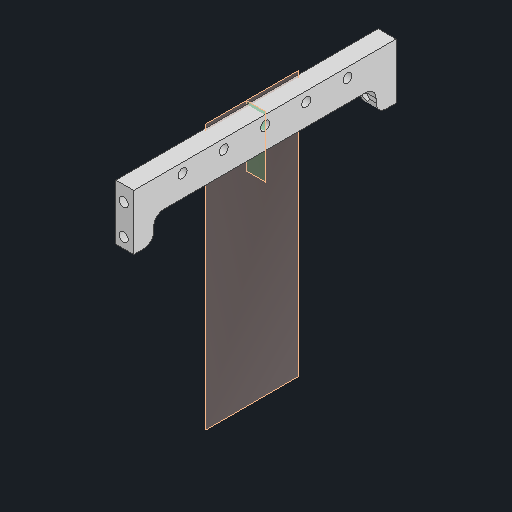
# Autodesk Inventor part: pci_slot_adapter_01
Saved by Autodesk Inventor 2022 (Build 260153000, 153)
## iProperties
Created: 2025-02-02
Part Number: pci_slot_adapter_01
Material: 一般
Document SubType Name: Modeling
Designer: nyxeon
Density: 1 g/cm^3
Appearance: 既定
Author: nyxeon
Autodesk Inventor part; units mm, degrees
ref_plane "YZ Plane" through (0, 0, 0) normal (1, 0, 0) x (0, 1, 0)
ref_plane "XZ Plane" through (0, 0, 0) normal (0, 1, 0) x (-1, 0, 0)
ref_plane "XY Plane" through (0, 0, 0) normal (0, 0, 1) x (1, 0, 0)
ref_plane "作業平面1" through (247.124, 159, 65.625) normal (1, 0, 0) x (0, 1, 0)
sketch "スケッチ1" plane through (247.124, 159, 65.625) normal (1, 0, 0) x (0, 1, 0)
  line L0 (60.3482, -6.7165) -> (60.3482, -14.8665) construction
  arc A0 (59.1658, -16) -> (60.3482, -14.8665) centre (59.15, -14.8001) ccw construction
  line L1 (53.4901, -16) -> (59.1658, -16) construction
  arc A1 (53.4901, -16) -> (53.2698, -16.0957) centre (53.4895, -16.3) ccw construction
  arc A2 (60.3482, -6.7165) -> (59.15, -5.583) centre (59.15, -6.783) ccw construction
  line L2 (59.15, -5.583) -> (53.4743, -5.583) construction
  line L3 (53.2621, -5.4951) -> (49.3015, -1.5345) construction
  arc A3 (53.2621, -5.4951) -> (53.4743, -5.583) centre (53.4743, -5.283) ccw construction
  arc A4 (48.95, -0.6859) -> (49.3015, -1.5345) centre (50.15, -0.6859) ccw construction
  arc A5 (49.3015, 0.2515) -> (48.95, -0.5971) centre (50.15, -0.5971) ccw construction
  line L4 (48.95, -0.6859) -> (48.95, -0.5971) construction
  line L5 (49.3015, 0.2515) -> (53.2621, 4.2121) construction
  arc A6 (53.4743, 4.3) -> (53.2621, 4.2121) centre (53.4743, 4) ccw construction
  line L6 (53.4743, 4.3) -> (59.15, 4.3) construction
  arc A7 (59.15, 4.3) -> (60.35, 5.5) centre (59.15, 5.5) ccw construction
  line L7 (60.35, 13.65) -> (60.35, 5.5) construction
  arc A8 (60.35, 13.65) -> (59.15, 14.85) centre (59.15, 13.65) ccw construction
  line L8 (59.15, 14.85) -> (53.4743, 14.85) construction
  arc A9 (53.2621, 14.9379) -> (53.4743, 14.85) centre (53.4743, 15.15) ccw construction
  line L9 (58.1, -68.625) -> (53.9, -68.625) construction
  line L10 (43.1, -68.625) -> (38.9, -68.625) construction
  line L11 (41, -68.625) -> (41, 67.375) construction
  line L12 (56, -68.625) -> (56, 67.375) construction
  line L13 (60.3482, -10.7915) -> (50.15, -10.7915) construction
  line L14 (60.35, 9.575) -> (50.15, 9.575) construction
  arc A10 (49.3015, -20.0486) -> (48.95, -20.8972) centre (50.15, -20.8972) ccw construction
  arc A11 (48.95, -20.986) -> (49.3015, -21.8346) centre (50.15, -20.986) ccw construction
  line L15 (48.95, -20.8972) -> (48.95, -20.986) construction
  line L16 (53.2698, -16.0957) -> (49.3015, -20.0486) construction
  line L17 (60.3482, 25.8665) -> (60.3482, 34.0165) construction
  arc A12 (60.3482, 34.0165) -> (59.1658, 35.15) centre (59.15, 33.9501) ccw construction
  line L18 (53.4901, 35.15) -> (59.1658, 35.15) construction
  arc A13 (53.2698, 35.2457) -> (53.4901, 35.15) centre (53.4895, 35.45) ccw construction
  arc A14 (59.15, 24.733) -> (60.3482, 25.8665) centre (59.15, 25.933) ccw construction
  line L19 (59.15, 24.733) -> (53.4743, 24.733) construction
  line L20 (53.2621, 24.6451) -> (49.3015, 20.6845) construction
  arc A15 (53.4743, 24.733) -> (53.2621, 24.6451) centre (53.4743, 24.433) ccw construction
  arc A16 (49.3015, 20.6845) -> (48.95, 19.8359) centre (50.15, 19.8359) ccw construction
  arc A17 (48.95, 19.7471) -> (49.3015, 18.8985) centre (50.15, 19.7471) ccw construction
  line L21 (48.95, 19.8359) -> (48.95, 19.7471) construction
  line L22 (49.3015, 18.8985) -> (53.2621, 14.9379) construction
  arc A18 (48.95, 40.0472) -> (49.3015, 39.1986) centre (50.15, 40.0472) ccw construction
  arc A19 (49.3015, 40.9846) -> (48.95, 40.136) centre (50.15, 40.136) ccw construction
  line L23 (48.95, 40.0472) -> (48.95, 40.136) construction
  line L24 (53.2698, 35.2457) -> (49.3015, 39.1986) construction
  line L25 (60.3482, 29.9415) -> (50.15, 29.9415) construction
  line L26 (60.3482, 66.5996) -> (60.3482, 74.7496) construction
  arc A20 (60.3482, 74.7496) -> (59.1658, 75.8831) centre (59.15, 74.6832) ccw construction
  line L27 (53.4901, 75.8831) -> (59.1658, 75.8831) construction
  arc A21 (53.2698, 75.9787) -> (53.4901, 75.8831) centre (53.4895, 76.1831) ccw construction
  arc A22 (59.15, 65.4661) -> (60.3482, 66.5996) centre (59.15, 66.6661) ccw construction
  line L28 (59.15, 65.4661) -> (53.4743, 65.4661) construction
  line L29 (53.2621, 65.3782) -> (49.3015, 61.4175) construction
  arc A23 (53.4743, 65.4661) -> (53.2621, 65.3782) centre (53.4743, 65.1661) ccw construction
  arc A24 (49.3015, 61.4175) -> (48.95, 60.569) centre (50.15, 60.569) ccw construction
  arc A25 (48.95, 60.4801) -> (49.3015, 59.6316) centre (50.15, 60.4801) ccw construction
  line L30 (48.95, 60.569) -> (48.95, 60.4801) construction
  line L31 (49.3015, 59.6316) -> (53.2621, 55.671) construction
  arc A26 (53.2621, 55.671) -> (53.4743, 55.5831) centre (53.4743, 55.8831) ccw construction
  line L32 (53.4743, 55.5831) -> (59.15, 55.5831) construction
  arc A27 (60.35, 54.3831) -> (59.15, 55.5831) centre (59.15, 54.3831) ccw construction
  line L33 (60.35, 46.2331) -> (60.35, 54.3831) construction
  arc A28 (59.15, 45.0331) -> (60.35, 46.2331) centre (59.15, 46.2331) ccw construction
  line L34 (59.15, 45.0331) -> (53.4743, 45.0331) construction
  arc A29 (53.4743, 45.0331) -> (53.2621, 44.9452) centre (53.4743, 44.7331) ccw construction
  arc A30 (48.95, 80.7802) -> (49.3015, 79.9317) centre (50.15, 80.7802) ccw construction
  arc A31 (49.3015, 81.7176) -> (48.95, 80.8691) centre (50.15, 80.8691) ccw construction
  line L35 (48.95, 80.7802) -> (48.95, 80.8691) construction
  line L36 (53.2698, 75.9787) -> (49.3015, 79.9317) construction
  line L37 (49.3015, 40.9846) -> (53.2621, 44.9452) construction
  line L38 (49.3015, -21.8346) -> (53.2621, -25.7952) construction
  arc A32 (53.2621, -25.7952) -> (53.4743, -25.8831) centre (53.4743, -25.5831) ccw construction
  line L39 (53.4743, -25.8831) -> (59.15, -25.8831) construction
  arc A33 (60.35, -27.0831) -> (59.15, -25.8831) centre (59.15, -27.0831) ccw construction
  line L40 (60.35, -35.2331) -> (60.35, -27.0831) construction
  arc A34 (59.15, -36.4331) -> (60.35, -35.2331) centre (59.15, -35.2331) ccw construction
  line L41 (59.15, -36.4331) -> (53.4743, -36.4331) construction
  arc A35 (53.4743, -36.4331) -> (53.2621, -36.521) centre (53.4743, -36.7331) ccw construction
  line L42 (49.3015, -40.4816) -> (53.2621, -36.521) construction
  arc A36 (49.3015, -40.4816) -> (48.95, -41.3301) centre (50.15, -41.3301) ccw construction
  line L43 (48.95, -41.419) -> (48.95, -41.3301) construction
  arc A37 (48.95, -41.419) -> (49.3015, -42.2675) centre (50.15, -41.419) ccw construction
  line L44 (53.2621, -46.2282) -> (49.3015, -42.2675) construction
  arc A38 (53.2621, -46.2282) -> (53.4743, -46.3161) centre (53.4743, -46.0161) ccw construction
  line L45 (59.15, -46.3161) -> (53.4743, -46.3161) construction
  arc A39 (60.3482, -47.4496) -> (59.15, -46.3161) centre (59.15, -47.5161) ccw construction
  line L46 (60.3482, -47.4496) -> (60.3482, -55.5996) construction
  arc A40 (59.1658, -56.7331) -> (60.3482, -55.5996) centre (59.15, -55.5332) ccw construction
  line L47 (53.4901, -56.7331) -> (59.1658, -56.7331) construction
  arc A41 (53.4901, -56.7331) -> (53.2698, -56.8287) centre (53.4895, -57.0331) ccw construction
  line L48 (53.2698, -56.8287) -> (49.3015, -60.7817) construction
  arc A42 (49.3015, -60.7817) -> (48.95, -61.6302) centre (50.15, -61.6302) ccw construction
  line L49 (48.95, -61.6302) -> (48.95, -61.7191) construction
  arc A43 (48.95, -61.7191) -> (49.3015, -62.5676) centre (50.15, -61.7191) ccw construction
  line L50 (49.3015, -62.5676) -> (53.2621, -66.5283) construction
  arc A44 (53.2621, -66.5283) -> (53.4743, -66.6162) centre (53.4743, -66.3162) ccw construction
  line L51 (59.15, -66.6162) -> (53.4743, -66.6162) construction
  arc A45 (60.35, -67.8162) -> (59.15, -66.6162) centre (59.15, -67.8162) ccw construction
  line L52 (60.35, -67.8162) -> (60.35, -75.9662) construction
  arc A46 (59.15, -77.1662) -> (60.35, -75.9662) centre (59.15, -75.9662) ccw construction
  line L53 (53.4743, -77.1662) -> (59.15, -77.1662) construction
  arc A47 (53.4743, -77.1662) -> (53.2621, -77.254) centre (53.4743, -77.4662) ccw construction
  line L54 (49.3015, -81.2147) -> (53.2621, -77.254) construction
  arc A48 (49.3015, -81.2147) -> (48.95, -82.0632) centre (50.15, -82.0632) ccw construction
  line L55 (48.95, -82.1521) -> (48.95, -82.0632) construction
  arc A49 (48.95, -82.1521) -> (49.3015, -83.0006) centre (50.15, -82.1521) ccw construction
  line L56 (53.2621, -86.9613) -> (49.3015, -83.0006) construction
  arc A50 (49.4429, 81.5762) -> (49.15, 80.8691) centre (50.15, 80.8691) ccw
  line L57 (49.15, 80.8691) -> (49.15, 80.7802)
  arc A51 (49.15, 80.7802) -> (49.4443, 80.0718) centre (50.15, 80.7802) ccw
  line L58 (49.4443, 80.0718) -> (53.4144, 76.117)
  arc A52 (53.4144, 76.117) -> (53.4897, 76.0831) centre (53.4895, 76.1831) ccw
  line L59 (53.4897, 76.0831) -> (59.1671, 76.0831)
  arc A53 (60.5482, 74.755) -> (59.1671, 76.0831) centre (59.15, 74.6832) ccw
  line L60 (60.5482, 74.755) -> (60.5482, 66.7378)
  arc A54 (59.15, 65.2661) -> (60.5482, 66.7378) centre (59.15, 66.6661) ccw
  line L61 (59.15, 65.2661) -> (53.4743, 65.2661)
  arc A55 (53.4743, 65.2661) -> (53.4036, 65.2368) centre (53.4743, 65.1661) ccw
  line L62 (53.4036, 65.2368) -> (49.4429, 61.2761)
  arc A56 (49.4429, 61.2761) -> (49.15, 60.569) centre (50.15, 60.569) ccw
  line L63 (49.15, 60.569) -> (49.15, 60.4801)
  arc A57 (49.15, 60.4801) -> (49.4429, 59.773) centre (50.15, 60.4801) ccw
  line L64 (49.4429, 59.773) -> (53.4036, 55.8124)
  arc A58 (53.4036, 55.8124) -> (53.4743, 55.7831) centre (53.4743, 55.8831) ccw
  line L65 (53.4743, 55.7831) -> (59.15, 55.7831)
  arc A59 (60.55, 54.3831) -> (59.15, 55.7831) centre (59.15, 54.3831) ccw
  line L66 (60.55, 54.3831) -> (60.55, 46.2331)
  arc A60 (59.15, 44.8331) -> (60.55, 46.2331) centre (59.15, 46.2331) ccw
  line L67 (59.15, 44.8331) -> (53.4743, 44.8331)
  arc A61 (53.4743, 44.8331) -> (53.4036, 44.8038) centre (53.4743, 44.7331) ccw
  line L68 (53.4036, 44.8038) -> (49.4429, 40.8431)
  arc A62 (49.4429, 40.8431) -> (49.15, 40.136) centre (50.15, 40.136) ccw
  line L69 (49.15, 40.136) -> (49.15, 40.0472)
  arc A63 (49.15, 40.0472) -> (49.4443, 39.3387) centre (50.15, 40.0472) ccw
  line L70 (49.4443, 39.3387) -> (53.4144, 35.384)
  arc A64 (53.4144, 35.384) -> (53.4897, 35.35) centre (53.4895, 35.45) ccw
  line L71 (53.4897, 35.35) -> (59.1671, 35.35)
  arc A65 (60.5482, 34.0219) -> (59.1671, 35.35) centre (59.15, 33.9501) ccw
  line L72 (60.5482, 34.0219) -> (60.5482, 26.0047)
  arc A66 (59.15, 24.533) -> (60.5482, 26.0047) centre (59.15, 25.933) ccw
  line L73 (59.15, 24.533) -> (53.4743, 24.533)
  arc A67 (53.4743, 24.533) -> (53.4036, 24.5037) centre (53.4743, 24.433) ccw
  line L74 (53.4036, 24.5037) -> (49.4429, 20.543)
  arc A68 (49.4429, 20.543) -> (49.15, 19.8359) centre (50.15, 19.8359) ccw
  line L75 (49.15, 19.8359) -> (49.15, 19.7471)
  arc A69 (49.15, 19.7471) -> (49.4429, 19.0399) centre (50.15, 19.7471) ccw
  line L76 (49.4429, 19.0399) -> (53.4036, 15.0793)
  arc A70 (53.4036, 15.0793) -> (53.4743, 15.05) centre (53.4743, 15.15) ccw
  line L77 (53.4743, 15.05) -> (59.15, 15.05)
  arc A71 (60.55, 13.65) -> (59.15, 15.05) centre (59.15, 13.65) ccw
  line L78 (60.55, 13.65) -> (60.55, 5.5)
  arc A72 (59.15, 4.1) -> (60.55, 5.5) centre (59.15, 5.5) ccw
  line L79 (59.15, 4.1) -> (53.4743, 4.1)
  arc A73 (53.4743, 4.1) -> (53.4036, 4.0707) centre (53.4743, 4) ccw
  line L80 (53.4036, 4.0707) -> (49.4429, 0.1101)
  arc A74 (49.4429, 0.1101) -> (49.15, -0.5971) centre (50.15, -0.5971) ccw
  line L81 (49.15, -0.5971) -> (49.15, -0.6859)
  arc A75 (49.15, -0.6859) -> (49.4429, -1.393) centre (50.15, -0.6859) ccw
  line L82 (49.4429, -1.393) -> (53.4036, -5.3537)
  arc A76 (53.4036, -5.3537) -> (53.4743, -5.383) centre (53.4743, -5.283) ccw
  line L83 (53.4743, -5.383) -> (59.15, -5.383)
  arc A77 (60.5482, -6.8547) -> (59.15, -5.383) centre (59.15, -6.783) ccw
  line L84 (60.5482, -6.8547) -> (60.5482, -14.8719)
  arc A78 (59.1671, -16.2) -> (60.5482, -14.8719) centre (59.15, -14.8001) ccw
  line L85 (59.1671, -16.2) -> (53.4897, -16.2)
  arc A79 (53.4897, -16.2) -> (53.4144, -16.234) centre (53.4895, -16.3) ccw
  line L86 (53.4144, -16.234) -> (49.4443, -20.1887)
  arc A80 (49.4443, -20.1887) -> (49.15, -20.8972) centre (50.15, -20.8972) ccw
  line L87 (49.15, -20.8972) -> (49.15, -20.986)
  arc A81 (49.15, -20.986) -> (49.4429, -21.6931) centre (50.15, -20.986) ccw
  line L88 (49.4429, -21.6931) -> (53.4036, -25.6538)
  arc A82 (53.4036, -25.6538) -> (53.4743, -25.6831) centre (53.4743, -25.5831) ccw
  line L89 (53.4743, -25.6831) -> (59.15, -25.6831)
  arc A83 (60.55, -27.0831) -> (59.15, -25.6831) centre (59.15, -27.0831) ccw
  line L90 (60.55, -27.0831) -> (60.55, -35.2331)
  arc A84 (59.15, -36.6331) -> (60.55, -35.2331) centre (59.15, -35.2331) ccw
  line L91 (59.15, -36.6331) -> (53.4743, -36.6331)
  arc A85 (53.4743, -36.6331) -> (53.4036, -36.6624) centre (53.4743, -36.7331) ccw
  line L92 (53.4036, -36.6624) -> (49.4429, -40.623)
  arc A86 (49.4429, -40.623) -> (49.15, -41.3301) centre (50.15, -41.3301) ccw
  line L93 (49.15, -41.3301) -> (49.15, -41.419)
  arc A87 (49.15, -41.419) -> (49.4429, -42.1261) centre (50.15, -41.419) ccw
  line L94 (49.4429, -42.1261) -> (53.4036, -46.0868)
  arc A88 (53.4036, -46.0868) -> (53.4743, -46.1161) centre (53.4743, -46.0161) ccw
  line L95 (53.4743, -46.1161) -> (59.15, -46.1161)
  arc A89 (60.5482, -47.5878) -> (59.15, -46.1161) centre (59.15, -47.5161) ccw
  line L96 (60.5482, -47.5878) -> (60.5482, -55.605)
  arc A90 (59.1671, -56.9331) -> (60.5482, -55.605) centre (59.15, -55.5332) ccw
  line L97 (59.1671, -56.9331) -> (53.4897, -56.9331)
  arc A91 (53.4897, -56.9331) -> (53.4144, -56.967) centre (53.4895, -57.0331) ccw
  line L98 (53.4144, -56.967) -> (49.4443, -60.9218)
  arc A92 (49.4443, -60.9218) -> (49.15, -61.6302) centre (50.15, -61.6302) ccw
  line L99 (49.15, -61.6302) -> (49.15, -61.7191)
  arc A93 (49.15, -61.7191) -> (49.4429, -62.4262) centre (50.15, -61.7191) ccw
  line L100 (49.4429, -62.4262) -> (53.4036, -66.3869)
  arc A94 (53.4036, -66.3869) -> (53.4743, -66.4162) centre (53.4743, -66.3162) ccw
  line L101 (53.4743, -66.4162) -> (59.15, -66.4162)
  arc A95 (60.55, -67.8162) -> (59.15, -66.4162) centre (59.15, -67.8162) ccw
  line L102 (60.55, -67.8162) -> (60.55, -75.9662)
  arc A96 (59.15, -77.3662) -> (60.55, -75.9662) centre (59.15, -75.9662) ccw
  line L103 (59.15, -77.3662) -> (53.4743, -77.3662)
  arc A97 (53.4743, -77.3662) -> (53.4036, -77.3955) centre (53.4743, -77.4662) ccw
  line L104 (53.4036, -77.3955) -> (49.4429, -81.3561)
  arc A98 (49.4429, -81.3561) -> (49.15, -82.0632) centre (50.15, -82.0632) ccw
  line L105 (49.15, -82.0632) -> (49.15, -82.1521)
  arc A99 (49.15, -82.1521) -> (49.4429, -82.8592) centre (50.15, -82.1521) ccw
  line L106 (49.4429, -82.8592) -> (53.454, -86.8703)
  line L107 (71, -65.625) -> (-359, -65.625) construction
  line L108 (52.6417, -65.625) -> (63.5, -65.625)
  line L109 (63.5, -65.625) -> (63.5, 64.375)
  line L110 (63.5, 64.375) -> (52.5418, 64.375)
  line L111 (71, 67.375) -> (-359, 67.375) construction
  line L112 (-359, 64.375) -> (71, 64.375) construction
  point P0 (-159, -65.625)
  dimension "d0" = 20.3
  dimension "d1" = 0.2
  dimension "d2" = 7.5
  dimension "d38" = 135
  dimension "d39" = 135
  constraints: 208 end point, 190 point on circle, 121 symmetric about line, 95 centre point, 7 vertical alignment, 5 equal length, 5 equal radius, 5 horizontal, 5 midpoint, 5 point on line, 5 tangent, 3 vertical, 139 other
  measures "d0" distance between parallel lines of L6 L1
  measures "d1" radial gap between concentric circles of A39 A89
  measures "d2" distance between parallel lines of L109 L12
  measures "d38" angle of L79 L80
  measures "d39" angle of L83 L82
extrude "押し出し1" add sketch "スケッチ1" against normal blind 1
sketch "スケッチ2" plane through (247.124, 159, 65.625) normal (1, 0, 0) x (0, 0, -1)
  line L0 (-60.569, 49.15) -> (-60.4801, 49.15) projected
  arc A0 (-60.4801, 49.15) -> (-59.773, 49.4429) centre (-60.4801, 50.15) ccw projected
  line L1 (-59.773, 49.4429) -> (-55.8124, 53.4036) projected
  arc A1 (-55.8124, 53.4036) -> (-55.7831, 53.4743) centre (-55.8831, 53.4743) ccw projected
  line L2 (-55.7831, 53.4743) -> (-55.7831, 59.15) projected
  arc A2 (-54.3831, 60.55) -> (-55.7831, 59.15) centre (-54.3831, 59.15) ccw projected
  line L3 (-54.3831, 60.55) -> (-46.2331, 60.55) projected
  arc A3 (-44.8331, 59.15) -> (-46.2331, 60.55) centre (-46.2331, 59.15) ccw projected
  line L4 (-44.8331, 59.15) -> (-44.8331, 53.4743) projected
  arc A4 (-44.8331, 53.4743) -> (-44.8038, 53.4036) centre (-44.7331, 53.4743) ccw projected
  line L5 (-44.8038, 53.4036) -> (-40.8431, 49.4429) projected
  arc A5 (-40.8431, 49.4429) -> (-40.136, 49.15) centre (-40.136, 50.15) ccw projected
  line L6 (-40.136, 49.15) -> (-40.0472, 49.15) projected
  arc A6 (-40.0472, 49.15) -> (-39.3387, 49.4443) centre (-40.0472, 50.15) ccw projected
  line L7 (-39.3387, 49.4443) -> (-35.384, 53.4144) projected
  arc A7 (-35.384, 53.4144) -> (-35.35, 53.4897) centre (-35.45, 53.4895) ccw projected
  line L8 (-35.35, 53.4897) -> (-35.35, 59.1671) projected
  arc A8 (-34.0219, 60.5482) -> (-35.35, 59.1671) centre (-33.9501, 59.15) ccw projected
  line L9 (-34.0219, 60.5482) -> (-26.0047, 60.5482) projected
  arc A9 (-24.533, 59.15) -> (-26.0047, 60.5482) centre (-25.933, 59.15) ccw projected
  line L10 (-24.533, 59.15) -> (-24.533, 53.4743) projected
  arc A10 (-24.533, 53.4743) -> (-24.5037, 53.4036) centre (-24.433, 53.4743) ccw projected
  line L11 (-24.5037, 53.4036) -> (-20.543, 49.4429) projected
  arc A11 (-20.543, 49.4429) -> (-19.8359, 49.15) centre (-19.8359, 50.15) ccw projected
  line L12 (-19.8359, 49.15) -> (-19.7471, 49.15) projected
  arc A12 (-19.7471, 49.15) -> (-19.0399, 49.4429) centre (-19.7471, 50.15) ccw projected
  line L13 (-19.0399, 49.4429) -> (-15.0793, 53.4036) projected
  arc A13 (-15.0793, 53.4036) -> (-15.05, 53.4743) centre (-15.15, 53.4743) ccw projected
  line L14 (-15.05, 53.4743) -> (-15.05, 59.15) projected
  arc A14 (-13.65, 60.55) -> (-15.05, 59.15) centre (-13.65, 59.15) ccw projected
  line L15 (-13.65, 60.55) -> (-5.5, 60.55) projected
  arc A15 (-4.1, 59.15) -> (-5.5, 60.55) centre (-5.5, 59.15) ccw projected
  line L16 (-4.1, 59.15) -> (-4.1, 53.4743) projected
  arc A16 (-4.1, 53.4743) -> (-4.0707, 53.4036) centre (-4, 53.4743) ccw projected
  line L17 (-4.0707, 53.4036) -> (-0.1101, 49.4429) projected
  arc A17 (-0.1101, 49.4429) -> (0.5971, 49.15) centre (0.5971, 50.15) ccw projected
  line L18 (0.5971, 49.15) -> (0.6859, 49.15) projected
  arc A18 (0.6859, 49.15) -> (1.393, 49.4429) centre (0.6859, 50.15) ccw projected
  line L19 (1.393, 49.4429) -> (5.3537, 53.4036) projected
  arc A19 (5.3537, 53.4036) -> (5.383, 53.4743) centre (5.283, 53.4743) ccw projected
  line L20 (5.383, 53.4743) -> (5.383, 59.15) projected
  arc A20 (6.8547, 60.5482) -> (5.383, 59.15) centre (6.783, 59.15) ccw projected
  line L21 (6.8547, 60.5482) -> (14.8719, 60.5482) projected
  arc A21 (16.2, 59.1671) -> (14.8719, 60.5482) centre (14.8001, 59.15) ccw projected
  line L22 (16.2, 59.1671) -> (16.2, 53.4897) projected
  arc A22 (16.2, 53.4897) -> (16.234, 53.4144) centre (16.3, 53.4895) ccw projected
  line L23 (16.234, 53.4144) -> (20.1887, 49.4443) projected
  arc A23 (20.1887, 49.4443) -> (20.8972, 49.15) centre (20.8972, 50.15) ccw projected
  line L24 (20.8972, 49.15) -> (20.986, 49.15) projected
  arc A24 (20.986, 49.15) -> (21.6931, 49.4429) centre (20.986, 50.15) ccw projected
  line L25 (21.6931, 49.4429) -> (25.6538, 53.4036) projected
  arc A25 (25.6538, 53.4036) -> (25.6831, 53.4743) centre (25.5831, 53.4743) ccw projected
  line L26 (25.6831, 53.4743) -> (25.6831, 59.15) projected
  arc A26 (27.0831, 60.55) -> (25.6831, 59.15) centre (27.0831, 59.15) ccw projected
  line L27 (27.0831, 60.55) -> (35.2331, 60.55) projected
  arc A27 (36.6331, 59.15) -> (35.2331, 60.55) centre (35.2331, 59.15) ccw projected
  line L28 (36.6331, 59.15) -> (36.6331, 53.4743) projected
  arc A28 (36.6331, 53.4743) -> (36.6624, 53.4036) centre (36.7331, 53.4743) ccw projected
  line L29 (36.6624, 53.4036) -> (40.623, 49.4429) projected
  arc A29 (40.623, 49.4429) -> (41.3301, 49.15) centre (41.3301, 50.15) ccw projected
  line L30 (41.3301, 49.15) -> (41.419, 49.15) projected
  arc A30 (41.419, 49.15) -> (42.1261, 49.4429) centre (41.419, 50.15) ccw projected
  line L31 (42.1261, 49.4429) -> (46.0868, 53.4036) projected
  arc A31 (46.0868, 53.4036) -> (46.1161, 53.4743) centre (46.0161, 53.4743) ccw projected
  line L32 (46.1161, 53.4743) -> (46.1161, 59.15) projected
  arc A32 (47.5878, 60.5482) -> (46.1161, 59.15) centre (47.5161, 59.15) ccw projected
  line L33 (47.5878, 60.5482) -> (55.605, 60.5482) projected
  arc A33 (56.9331, 59.1671) -> (55.605, 60.5482) centre (55.5332, 59.15) ccw projected
  line L34 (56.9331, 59.1671) -> (56.9331, 53.4897) projected
  arc A34 (56.9331, 53.4897) -> (56.967, 53.4144) centre (57.0331, 53.4895) ccw projected
  line L35 (56.967, 53.4144) -> (60.9218, 49.4443) projected
  arc A35 (60.9218, 49.4443) -> (61.6302, 49.15) centre (61.6302, 50.15) ccw projected
  line L36 (61.6302, 49.15) -> (61.7191, 49.15) projected
  arc A36 (61.7191, 49.15) -> (62.4262, 49.4429) centre (61.7191, 50.15) ccw projected
  line L37 (62.4262, 49.4429) -> (65.625, 52.6417) projected
  line L38 (65.625, 52.6417) -> (65.625, 63.5) projected
  line L39 (65.625, 63.5) -> (-64.375, 63.5) projected
  line L40 (-64.375, 63.5) -> (-64.375, 52.5418) projected
  line L41 (-64.375, 52.5418) -> (-61.2761, 49.4429) projected
  arc A37 (-61.2761, 49.4429) -> (-60.569, 49.15) centre (-60.569, 50.15) ccw projected
  point P0 (65.625, -159)
extrude "押し出し2" add sketch "スケッチ2" along normal blind 0.2
sketch "スケッチ3" plane through (247.324, 159, 65.625) normal (1, 0, 0) x (0, 0, -1)
  line L0 (68.625, 58.1) -> (68.625, 53.9) construction
  line L1 (65.625, 53.9) -> (65.625, 58.1) construction
  line L2 (68.625, 43.1) -> (68.625, 38.9) construction
  line L3 (65.625, 43.1) -> (65.625, 38.9) construction
  line L4 (-64.375, 43.1) -> (-64.375, 38.9) construction
  line L5 (-67.375, 38.9) -> (-67.375, 43.1) construction
  line L6 (-64.375, 58.1) -> (-64.375, 53.9) construction
  line L7 (-67.375, 53.9) -> (-67.375, 58.1) construction
  line L8 (61.6302, 49.15) -> (61.7191, 49.15) construction
  line L9 (-60.569, 49.15) -> (-60.4801, 49.15) construction
  line L10 (65.625, 36) -> (-64.375, 36)
  line L11 (65.625, 63.5) -> (-64.375, 63.5) projected
  line L12 (-64.375, 63.5) -> (65.625, 63.5) projected
  line L13 (65.625, 36) -> (65.625, 63.5)
  line L14 (-64.375, 52.5418) -> (-64.375, 63.5) projected
  line L15 (-64.375, 36) -> (-64.375, 63.5)
  point P0 (65.625, -159)
  point P1 (65.625, 41)
  dimension "d7" = 5
  constraints: 6 end point, 2 vertical, 1 horizontal, 1 midpoint
  measures "d7" distance from line of point (65.625, 41) L10
extrude "押し出し3" add sketch "スケッチ3" along normal blind 7.676
sketch "スケッチ4" plane through (246.124, 211.6417, 0) normal (0, 0, -1) x (-1, 0, 0)
  circle A0 centre (-3.876, -11.6417) radius 2.1 construction
  circle A1 centre (-3.876, 3.3583) radius 2.1 construction
  circle A2 centre (-3.876, -11.6417) radius 1.6
  circle A3 centre (-3.876, 3.3583) radius 1.6
  point P0 (246.124, -211.6417)
  dimension "d10" = 3.2
  constraints: 2 centre point, 2 coincident, 1 equal radius
  measures "d10" diameter of A2
extrude "押し出し4" cut sketch "スケッチ4" against normal blind 16
ref_plane "作業平面2" through (246.124, 211.6417, 65) normal (0, 0, -1) x (-1, 0, 0)
mirror "ミラー1" about plane through (246.124, 211.6417, 65) normal (0, 0, -1) of "押し出し4"
sketch "スケッチ5" plane through (246.124, 159, 65.625) normal (-1, 0, 0) x (0, 0, 1)
  line L0 (61.2761, 49.4429) -> (64.375, 52.5418) projected
  arc A0 (60.569, 49.15) -> (61.2761, 49.4429) centre (60.569, 50.15) ccw projected
  line L1 (60.4801, 49.15) -> (60.569, 49.15) projected
  line L2 (64.375, 52.5418) -> (64.375, 36) projected
  line L3 (64.375, 36) -> (-65.625, 36) projected
  line L4 (-65.625, 36) -> (-65.625, 52.6417) projected
  line L5 (-65.625, 52.6417) -> (-62.4262, 49.4429) projected
  arc A1 (-62.4262, 49.4429) -> (-61.7191, 49.15) centre (-61.7191, 50.15) ccw projected
  line L6 (-61.7191, 49.15) -> (-61.6302, 49.15) projected
  line L7 (-61.6747, 49.15) -> (-61.6747, 36)
  line L8 (60.5246, 49.15) -> (60.5246, 36)
  point P0 (-65.625, -159)
  constraints: 4 end point, 2 midpoint, 2 point on line, 1 perpendicular, 1 vertical
extrude "押し出し5" add sketch "スケッチ5" against normal up to surface (1.2 mm away)
sketch "スケッチ6" plane through (246.124, 159, 65.625) normal (-1, 0, 0) x (0, 0, 1)
  line L0 (4.1, 53.4743) -> (4.1, 59.15) construction
  line L1 (-5.383, 59.15) -> (-5.383, 53.4743) construction
  line L2 (64.375, 63.5) -> (-65.625, 63.5) construction
  circle A0 centre (-0.6415, 58.7585) radius 4.7415 construction
  line L3 (15.05, 59.15) -> (15.05, 53.4743) construction
  circle A1 centre (-0.6415, 58.7585) radius 2.25
  circle A2 centre (-21.0745, 58.7585) radius 2.25
  circle A3 centre (-41.5074, 58.7585) radius 2.25
  circle A4 centre (19.7915, 58.7585) radius 2.25
  circle A5 centre (-0.6415, 58.7585) radius 2.25
  circle A6 centre (-21.0745, 58.7585) radius 2.25
  circle A7 centre (40.2245, 58.7585) radius 2.25
  circle A8 centre (19.7915, 58.7585) radius 2.25
  circle A9 centre (-0.6415, 58.7585) radius 2.25
  point P0 (-65.625, -159)
  dimension "d16" = 20.433
  dimension "d17" = 4.5
  dimension "d20" = 20.433
  dimension "d23" = 20.433
  constraints: 10 centre point, 3 tangent, 2 horizontal, 1 coincident, 16 other
  measures "d16" distance between parallel lines of L1 L3
  measures "d17" diameter of A1
  measures "d20" distance of A1.centre A2.centre
  measures "d23" distance of A1.centre A4.centre
extrude "押し出し6" cut sketch "スケッチ6" against normal through all
sketch "スケッチ7" plane through (247.324, 159, 65.625) normal (-1, 0, 0) x (0, 0, 1)
  line L0 (60.5246, 36) -> (-61.6747, 36) construction
  line L1 (54.5246, 36) -> (-55.6747, 36)
  line L2 (-55.6747, 36) -> (-55.6747, 48)
  line L3 (-55.6747, 48) -> (54.5246, 48)
  line L4 (54.5246, 48) -> (54.5246, 36)
  line L5 (46.2331, 60.55) -> (54.3831, 60.55) construction
  point P0 (-65.625, -159)
  point P1 (-0.5751, 36)
  point P2 (50.3081, 60.55)
  dimension "d30" = 12
  dimension "d34" = 6
  constraints: 8 end point, 3 midpoint, 2 parallel, 1 horizontal, 1 perpendicular, 1 point on line
  measures "d30" distance between parallel lines of L3 L0
  measures "d34" distance from line of L4 L0.start
extrude "押し出し7" cut sketch "スケッチ7" against normal through all
fillet "フィレット3" radius 5 4 edges at (251.162, 195, 120.1496) (251.162, 207, 120.1496) (251.162, 207, 9.9503) (251.162, 195, 9.9503)
sketch "スケッチ8" plane through (246.124, 195, 130) normal (0, 0, 1) x (1, 0, 0)
  circle A0 centre (3.876, 5) radius 1.6 construction
  circle A1 centre (3.876, 20) radius 1.6 construction
  circle A2 centre (3.876, 5) radius 2.25
  circle A3 centre (3.876, 20) radius 2.25
  point P0 (-246.124, -195)
  dimension "d35" = 4.5
  constraints: 2 centre point, 2 coincident, 1 equal radius
  measures "d35" diameter of A2
extrude "押し出し8" cut sketch "スケッチ8" against normal blind 5
mirror "ミラー3" about plane through (246.124, 211.6417, 65) normal (0, 0, -1) of "押し出し8"
fillet "フィレット2" radius 1 2 edges at (246.724, 208.15, 126.1496) (246.724, 208.15, 3.9503)
equation "\"d39\" = d38"
equation "\"d20\" = d16"
equation "\"d23\" = d16"
